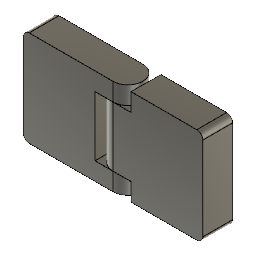
Hinge v1 (Autodesk Fusion 360 design; units mm, degrees)
Autodesk Fusion 360 part; units mm, degrees
sketch "Sketch2" plane through (0, 0, 0) normal (0, 0, 1) x (1, 0, 0)
  line L0 (-15, 0) -> (0, 0)
  line L1 (0, 5) -> (-15, 5)
  line L2 (-15, 5) -> (-15, 0)
  arc A0 (0, 0) -> (0, 5) centre (0, 2.5) ccw
  circle A1 centre (0, 2.5) radius 1.75
  circle A2 centre (0, 2.5) radius 1.45
  line L3 (-3, 5) -> (-3, 0)
  dimension "d1" = 15
  dimension "d2" = 5
  dimension "d3" = 3.5
  dimension "d4" = 2.9
  dimension "d5" = 12
  constraint horizontal L0
  constraint horizontal L1
  constraint vertical L2
  constraint coincident L0.end A0
  constraint tangent L0 A0
  constraint tangent L1 A0
  constraint concentric A0 A1
  constraint concentric A0 A2
  constraint coincident L1 L3.start
  constraint perpendicular L1 L3
  measures "d1" distance of L1.start L1.end
  measures "d2" distance of L0.start L1.end
  measures "d3" diameter of A1
  measures "d4" diameter of A2
  measures "d5" distance of L2 L3
extrude "Extrude1" add sketch "Sketch2" along normal blind 3 contours L0 L1 L2 L3 | L0 L1 A0 L3 | A1 | A2 makes body 1
extrude "Extrude2" add sketch "Sketch2" along normal blind 8 contours L0 L1 L2 L3 | A2 bodies 1
ref_plane "WorkPlane1" through (0, 2.5, 8) normal (0, 0, 1) x (1, 0, 0)
mirror "Mirror1" about plane through (0, 2.5, 8) normal (0, 0, 1) of bodies 1 merged
copy_body "Body->Comp1" bodies 1 removing the originals makes body 2 in component "Component"
extrude "Extrude3" add sketch "Sketch2" along normal blind 10 separate body contours L0 L1 L2 L3 | L0 L1 A0 L3 makes body 3
extrude "Extrude4" add sketch "Sketch2" against normal blind 3 separate body contours L0 L1 L2 L3 makes body 4
ref_plane "WorkPlane2" through (-6.25, 2.5, 5) normal (0, 0, 1) x (1, 0, 0)
mirror "Mirror2" about plane through (-6.25, 2.5, 5) normal (0, 0, 1) of bodies 4 makes body 5
combine "Combine1" operation add target body 3 tool bodies 5 4
copy_body "Body->Comp2" bodies 3 removing the originals makes body 6 in component "Component'"
move_body "Move1" bodies 2 to x (1, 0, 0) y (0, 1, 0) z (0, 0, 1) at (10, -40, 18) in component "Component"
fillet "Fillet1" radius 1 2 edges at (-15, 2.5, 13) (-15, 2.5, -3) on bodies 6 in component "Component'"
fillet "Fillet1'" radius 1 2 edges at (-5, -37.5, 18) (-5, -37.5, 34) on bodies 2 in component "Component"
component "Component" placed x (1, 0, 0) y (0, 1, 0) z (0, 0, 1) at (0, 0, 0)
component "Component'" placed x (1, 0, 0) y (0, 1, 0) z (0, 0, 1) at (10, -40, 21)
equation "d4 = d3 - ( 2 * 0.3 ) * 1 mm"
